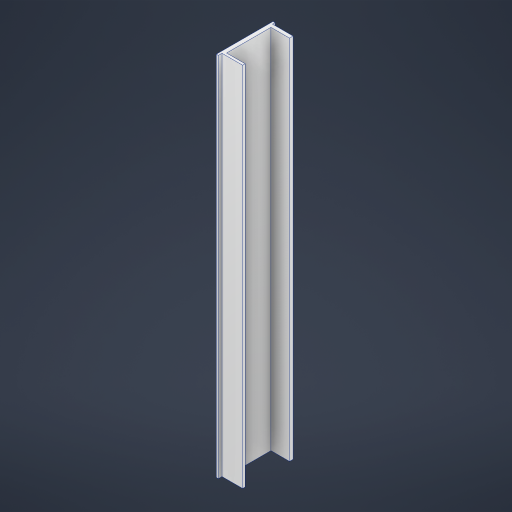
# Autodesk Inventor part: YKrep
Saved by Autodesk Inventor 2024 (Build 280153000, 153)
## iProperties
Created: 2023-06-19
Part Number: YKrep
Material: Aluminum 6061
Document SubType Name: Modeling
Designer: KirikDK
Mass: 2426.5 g
Surface Area: 2727.08 cm^2
Volume: 898.704 cm^3
Density: 2.7 g/cm^3
Appearance: Aluminum - Flat
Author: KirikDK
Autodesk Inventor part; units mm, degrees
ref_plane "YZ Plane" through (0, 0, 0) normal (1, 0, 0) x (0, 1, 0)
ref_plane "XZ Plane" through (0, 0, 0) normal (0, 1, 0) x (-1, 0, 0)
ref_plane "XY Plane" through (0, 0, 0) normal (0, 0, 1) x (1, 0, 0)
sketch "Sketch1" plane through (0, 0, 0) normal (0, 1, 0) x (-1, 0, 0)
  line L0 (20, 40) -> (-33.4783, 40)
  line L1 (-33.4783, 40) -> (-33.4783, -70)
  line L2 (-33.4783, -70) -> (20, -70)
  line L3 (20, -70) -> (20, 40)
  line L4 (16, 40) -> (16, 33)
  line L5 (16, 33) -> (-24, 33)
  line L6 (-24, 33) -> (-24, 28)
  line L7 (-24, 28) -> (12, 28)
  line L8 (12, 28) -> (12, -58)
  line L9 (12, -58) -> (-24, -58)
  line L10 (-24, -58) -> (-24, -65)
  line L11 (-24, -65) -> (16, -65)
  line L12 (16, -65) -> (16, -70)
  point P0 (0, 0)
  dimension "d0" = 110
  constraints: 26 end point, 7 perpendicular, 6 point on line, 2 parallel, 1 horizontal, 1 vertical
  measures "d0" distance of L2.end L0.start
extrude "Extrusion1" add sketch "Sketch1" along normal blind 711 contours L3 L2 L12 L11 L10 L9 L8 L7 L6 L5 L4 L0
body "Solid1"
